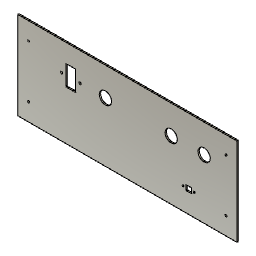
Control box front (Autodesk Fusion 360 design; units mm, degrees)
Autodesk Fusion 360 part; units mm, degrees
sketch "Panel" plane through (0, 0, 0) normal (0, 1, 0) x (1, 0, 0)
  line L0 (250, -18) -> (250, -13)
  circle A0 centre (175, -148) radius 14
  line L1 (-140, -125) -> (-118, -171) construction
  circle A1 centre (-108, -148) radius 2.5
  circle A2 centre (152.5, -63) radius 2
  line L2 (140, -80) -> (140, -13) construction
  line L3 (-140, -125) -> (-140, -171)
  line L4 (123.1713, -63) -> (203.1713, -63) construction
  line L5 (-118, -125) -> (-140, -171) construction
  line L6 (250, -13) -> (-250, -13)
  line L7 (250, -213) -> (250, -13)
  circle A3 centre (100, -148) radius 14
  circle A4 centre (-150, -148) radius 2.5
  line L8 (-118, -171) -> (-118, -125)
  circle A5 centre (-50, -148) radius 14
  line L9 (-250, -213) -> (250, -213)
  line L10 (-250, -13) -> (-250, -213)
  line L11 (250, -13) -> (-250, -13)
  circle A6 centre (225, -53) radius 2.25
  line L12 (225, -213) -> (225, -13) construction
  line L13 (-140, -171) -> (-118, -171)
  line L14 (-118, -125) -> (-140, -125)
  line L15 (250, -148) -> (-250, -148) construction
  line L16 (-225, -213) -> (-225, -13) construction
  circle A7 centre (225, -173) radius 2.25
  circle A8 centre (-225, -53) radius 2.25
  circle A9 centre (-225, -173) radius 2.25
  circle A10 centre (126.8597, -63) radius 2
  line L17 (146.25, -57.25) -> (133.75, -57.25)
  line L18 (133.75, -57.25) -> (133.75, -68.75)
  line L19 (133.75, -68.75) -> (146.25, -68.75)
  line L20 (146.25, -68.75) -> (146.25, -57.25)
  line L21 (146.25, -57.25) -> (133.75, -68.75) construction
  line L22 (133.75, -57.25) -> (146.25, -68.75) construction
  point P0 (189, -148)
  point P1 (-152.5, -148)
  point P2 (-129, -148)
  point P3 (140, -63)
  dimension "d1" = 500
  dimension "d2" = 200
  dimension "d3" = 28
  dimension "d4" = 28
  dimension "d5" = 28
  dimension "d6" = 150
  dimension "d7" = 46
  dimension "d8" = 22
  dimension "d9" = 5
  dimension "d10" = 5
  dimension "d11" = 21
  dimension "d12" = 21
  dimension "d13" = 100
  dimension "d14" = 75
  dimension "d15" = 25
  dimension "d16" = 25
  dimension "d17" = 4.5
  dimension "d18" = 40
  dimension "d25" = 110
  dimension "d28" = 4
  dimension "d30" = 12.5
  dimension "d32" = 50
  dimension "d34" = 13
  dimension "d35" = 75
  dimension "d36" = 250
  dimension "d37" = 65
  dimension "d38" = 4.5
  dimension "d39" = 4.5
  dimension "d40" = 4.5
  dimension "d41" = 40
  dimension "d42" = 40
  dimension "d43" = 40
  dimension "d44" = 4
  dimension "d45" = 12.5
  constraint coincident L0.end L6.start
  constraint coincident L15.start L7
  constraint coincident L15.end L10
  constraint perpendicular L10 L15
  constraint coincident A0.centre L15
  constraint coincident A3.centre L15
  constraint coincident A5.centre L15
  constraint perpendicular L3 L14
  constraint parallel L13 L14
  constraint parallel L3 L8
  constraint coincident P2 L5
  constraint coincident P2 L1
  constraint coincident P2 L15
  constraint coincident A1.centre L15
  constraint coincident A4.centre L15
  constraint coincident P0 L15
  constraint coincident P0 A0
  constraint coincident P1 A4
  constraint coincident P1 L15
  constraint coincident L16.start L9
  constraint coincident L16.end L11
  constraint perpendicular L11 L16
  constraint coincident L12.start L9
  constraint coincident L12.end L11
  constraint perpendicular L11 L12
  constraint coincident A6.centre L12
  constraint coincident L2.end L11
  constraint perpendicular L2 L11
  constraint perpendicular L2 L4
  constraint coincident A2.centre L4
  constraint coincident L12 A7.centre
  constraint coincident L16 A8.centre
  constraint coincident L16 A9.centre
  constraint equal L6 L9
  constraint horizontal L9
  constraint horizontal L6
  constraint coincident L4 A10.centre
  constraint horizontal L17
  constraint perpendicular L17 L18
  constraint parallel L17 L19
  constraint parallel L18 L20
  constraint coincident L21 P3
  constraint coincident L22 P3
  constraint coincident L2 P3
  constraint coincident L4 P3
  measures "d1" distance of L0.end L6.end
  measures "d2" distance of L0.end L7.start
  measures "d4" diameter of A3
  measures "d5" diameter of A5
  measures "d6" distance of A3.centre A5.centre
  measures "d7" distance of L1.start L3.end
  measures "d8" distance of L3.end L1.end
  measures "d9" diameter of A1
  measures "d10" diameter of A4
  measures "d11" distance of P2 A4.centre
  measures "d12" distance of P2 A1.centre
  measures "d13" distance of A4.centre L10
  measures "d14" distance of A3.centre A0.centre
  measures "d15" distance of L10 L16
  measures "d16" distance of L7 L12
  measures "d17" diameter of A6
  measures "d18" distance of A6.centre L11
  measures "d25" distance of L2 L7
  measures "d28" diameter of A2
  measures "d30" distance of A2.centre L2
  measures "d32" distance of L4 L11
  measures "d34" distance of origin L11
  measures "d35" distance of A0.centre L7
  measures "d36" distance of origin L10
  measures "d37" distance of L9 L15
  measures "d39" diameter of A8
  measures "d40" diameter of A9
  measures "d41" distance of L6 A8.centre
  measures "d42" distance of L9 A7.centre
  measures "d43" distance of L9 A9.centre
  measures "d44" diameter of A10
  measures "d45" distance of L18.end L19.end
extrude "Extrude1" add sketch "Panel" along normal blind 3
equation "d4 = d3"
equation "d5 = d3"
equation "d6 = d140 * 2"
equation "d12 = d124"
equation "d18 = d41"
equation "d22 = d163"
equation "d36 = d1 / 2"
equation "d38 = d17"
equation "d39 = d17"
equation "d40 = d17"
equation "d42 = d41"
equation "d43 = d41"
equation "d44 = d28"
named bodies: "Panel"
